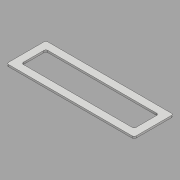
# Autodesk Inventor part: smaho_mount_board
Saved by Autodesk Inventor 2017 (Build 210142000, 142)
## iProperties
Part Number: smaho_mount_board
Material: 一般
Document SubType Name: Modeling
Designer: uhiit
Density: 1 g/cm^3
Appearance: 既定
Author: uhiit
Autodesk Inventor part; units mm, degrees
ref_plane "YZ Plane" through (0, 0, 0) normal (1, 0, 0) x (0, 1, 0)
ref_plane "XZ Plane" through (0, 0, 0) normal (0, 1, 0) x (-1, 0, 0)
ref_plane "XY Plane" through (0, 0, 0) normal (0, 0, 1) x (1, 0, 0)
sketch "スケッチ1" plane through (0, 0, 0) normal (0, 0, 1) x (1, 0, 0)
  line L0 (0, 0) -> (130, 0)
  line L1 (130, 0) -> (130, 40)
  line L2 (130, 40) -> (0, 40)
  line L3 (0, 40) -> (0, 0)
  dimension "d0" = 130
  dimension "d1" = 40
  constraints: 8 end point, 2 parallel, 1 horizontal, 1 perpendicular
  measures "d0" distance of L2.end L1.end
  measures "d1" distance of L1.end L0.end
extrude "押し出し1" add sketch "スケッチ1" along normal blind 2
sketch "スケッチ2" plane through (0, 0, 2) normal (0, 0, 1) x (1, 0, 0)
  line L0 (130, 40) -> (0, 40) projected
  line L1 (0, 40) -> (130, 40)
  line L2 (130, 40) -> (130, 0)
  line L3 (130, 0) -> (0, 0)
  line L4 (0, 0) -> (0, 40)
  line L5 (7.5, 7.5) -> (122.5, 7.5)
  line L6 (122.5, 7.5) -> (122.5, 32.5)
  line L7 (122.5, 32.5) -> (7.5, 32.5)
  line L8 (7.5, 32.5) -> (7.5, 7.5)
  dimension "d4" = 7.5
  constraints: 16 end point, 4 parallel, 2 perpendicular, 1 horizontal, 3 other
  measures "d4" distance between parallel lines of L3 L5
extrude "押し出し2" cut sketch "スケッチ2" against normal blind 2 contours L8 L7 L6 L5
fillet "フィレット1" radius 2 8 edges at (0, 40, 1) (0, 0, 1) (7.5, 7.5, 1) (7.5, 32.5, 1) (130, 40, 1) (130, 0, 1) (122.5, 7.5, 1) (122.5, 32.5, 1)
